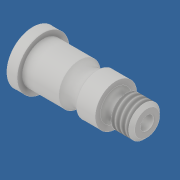
# Autodesk Inventor part: Öler
Saved by Autodesk Inventor 2018 (Build 220112000, 112)
## iProperties
Created: 2018-10-23
Part Number: Öler
Material: Generisch
Document SubType Name: Modeling
Designer: M.Knabel
Density: 1 g/cm^3
Appearance: Vorgabe
Author: M.Knabel
Autodesk Inventor part; units mm, degrees
ref_plane "YZ Plane" through (0, 0, 0) normal (1, 0, 0) x (0, 1, 0)
ref_plane "XZ Plane" through (0, 0, 0) normal (0, 1, 0) x (-1, 0, 0)
ref_plane "XY Plane" through (0, 0, 0) normal (0, 0, 1) x (1, 0, 0)
sketch "Skizze1" plane through (0, 0, 0) normal (0, 0, 1) x (1, 0, 0)
  line L0 (0, -1.0072) -> (0, 6.0435) projected
  line L1 (-2.2, 0) -> (13.2, 0) projected
  line L2 (0, 2.5) -> (0, 1.75)
  line L3 (0, 2.5) -> (1, 2.5)
  line L4 (1, 2.5) -> (1, 2)
  line L5 (1, 2) -> (4.5, 2)
  line L6 (0, 1.75) -> (4, 1.75)
  arc A0 (4.5, 2) -> (6.1971, 2) centre (5.3485, 2.7) ccw
  line L7 (6.1971, 2) -> (8, 2)
  line L8 (8, 2) -> (8, 1.5)
  arc A1 (8, 1.5) -> (9, 1.5) centre (8.5, 1.5) ccw
  line L9 (9, 1.5) -> (11, 1.5)
  line L10 (11, 1.5) -> (11, 0.65)
  line L11 (11, 0.65) -> (4.923, 0.65)
  line L12 (4.923, 0.65) -> (4, 1.75)
  line L13 (5.3485, 5.0362) -> (5.3485, 0.3638) construction
  point P0 (0, 0)
  dimension "d0" = 4
  dimension "d1" = 5
  dimension "d2" = 3.5
  dimension "d3" = 4
  dimension "d4" = 1.3
  dimension "d6" = 6.5
  dimension "d7" = 0.5
  dimension "d8" = 3
  dimension "d9" = 3
  dimension "d10" = 11
  dimension "d11" = 1
  dimension "d13" = 3.2
  dimension "d14" = 1.1
  dimension "d15" = 130
  constraints: 24 end point, 5 perpendicular, 4 horizontal, 4 point on circle, 4 point on line, 2 centre point, 1 coincident, 1 midpoint, 1 symmetric about line, 1 tangent, 1 vertical
  measures "d0" distance from line of L6.end L0
  measures "d1" diameter of L3 L1
  measures "d2" diameter of L6 L1
  measures "d3" diameter of L5 L1
  measures "d4" diameter of L11 L1
  measures "d6" distance from line of L10 L5.end
  measures "d7" radius of A1
  measures "d8" distance between parallel lines of L8 L10
  measures "d9" diameter of L9 L1
  measures "d10" distance between parallel lines of L10 L0
  measures "d11" distance between parallel lines of L0 L4
  measures "d14" radius of A0
  measures "d15" angle of L1 L12
revolve "Umdrehung1" add sketch "Skizze1" angle 360 about axis through (-10, 0, 0) along (1, 0, 0)
thread "Gewinde1" size "M3x0.5" class "6g" standard "ANSI Metric M Profile" full length
chamfer "Fase1" distance 0.3 angle 45 1 edges at (11, -1.5, 0)
